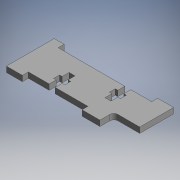
# Autodesk Inventor part: Part14
Saved by Autodesk Inventor 2019.2 (Build 232265000, 265)
## iProperties
Part Number: Part14
Material: Generic
Document SubType Name: Modeling
Designer: richard.girt
Mass: 2.90152 g
Surface Area: 27.0963 cm^2
Volume: 2.90152 cm^3
Density: 1 g/cm^3
Appearance: Default
Author: richard.girt
Autodesk Inventor part; units mm, degrees
ref_plane "YZ Plane" through (0, 0, 0) normal (1, 0, 0) x (0, 1, 0)
ref_plane "XZ Plane" through (0, 0, 0) normal (0, 1, 0) x (-1, 0, 0)
ref_plane "XY Plane" through (0, 0, 0) normal (0, 0, 1) x (1, 0, 0)
sketch "Sketch1" plane through (0, 0, 0) normal (0, 1, 0) x (-1, 0, 0)
  line L0 (-30, -12) -> (30, -12)
  line L1 (30, -12) -> (30, 12)
  line L2 (30, 12) -> (-30, 12)
  line L3 (-30, 12) -> (-30, -12)
  line L4 (-30, -12) -> (30, 12) construction
  line L5 (30, -12) -> (-30, 12) construction
  line L6 (25, -12) -> (-22, -12)
  line L7 (-22, -12) -> (-22, -9)
  line L8 (-22, -9) -> (25, -9)
  line L9 (25, -9) -> (25, -12)
  line L10 (22, 12) -> (-8, 12)
  line L11 (-8, 12) -> (-8, 9)
  line L12 (-8, 9) -> (22, 9)
  line L13 (22, 9) -> (22, 12)
  line L14 (-30, 12) -> (-17, 12)
  line L15 (-17, 12) -> (-17, 7)
  line L16 (-19, 5) -> (-30, 5)
  line L17 (-30, 5) -> (-30, 12)
  line L18 (11.75, -1) -> (8.25, -1)
  line L19 (8.25, -1) -> (8.25, 9)
  line L20 (8.25, 9) -> (11.75, 9)
  line L21 (11.75, 9) -> (11.75, -1)
  line L22 (11.75, -1) -> (8.25, 9) construction
  line L23 (8.25, -1) -> (11.75, 9) construction
  line L24 (12.8, 5.5) -> (7.2, 5.5)
  line L25 (7.2, 5.5) -> (7.2, 2.5)
  line L26 (7.2, 2.5) -> (12.8, 2.5)
  line L27 (12.8, 2.5) -> (12.8, 5.5)
  line L28 (12.8, 5.5) -> (7.2, 2.5) construction
  line L29 (7.2, 5.5) -> (12.8, 2.5) construction
  line L30 (-8.25, -9) -> (-11.75, -9)
  line L31 (-11.75, -9) -> (-11.75, 1)
  line L32 (-11.75, 1) -> (-8.25, 1)
  line L33 (-8.25, 1) -> (-8.25, -9)
  line L34 (-8.25, -9) -> (-11.75, 1) construction
  line L35 (-11.75, -9) -> (-8.25, 1) construction
  line L36 (-7.2, -2.5) -> (-12.8, -2.5)
  line L37 (-12.8, -2.5) -> (-12.8, -5.5)
  line L38 (-12.8, -5.5) -> (-7.2, -5.5)
  line L39 (-7.2, -5.5) -> (-7.2, -2.5)
  line L40 (-7.2, -2.5) -> (-12.8, -5.5) construction
  line L41 (-12.8, -2.5) -> (-7.2, -5.5) construction
  arc A0 (-19, 5) -> (-17, 7) centre (-19, 7) ccw
  point P0 (0, 0)
  point P1 (10, 4)
  point P2 (10, 4)
  point P3 (10, 9)
  point P4 (-10, -4)
  point P5 (-10, -4)
  point P6 (-10, 1)
  point P7 (-10, -9)
  dimension "d0" = 60
  dimension "d1" = 24
  dimension "d3" = 3
  dimension "d4" = 47
  dimension "d5" = 8
  dimension "d6" = 30
  dimension "d7" = 3
  dimension "d8" = 7
  dimension "d9" = 13
  dimension "d10" = 10
  dimension "d12" = 5.6
  dimension "d14" = 20
  dimension "d15" = 10
  dimension "d16" = 5.6
  dimension "d17" = 3.5
  dimension "d18" = 20
  dimension "d19" = 2
  dimension "d22" = 9
  dimension "d23" = 8
  dimension "d24" = 5
  dimension "d25" = 3
  constraints: 84 end point, 18 parallel, 15 midpoint, 8 horizontal, 8 perpendicular, 4 point on line, 2 point on circle, 2 tangent, 1 centre point
  measures "d0" distance of L0.start L0.end
  measures "d1" distance of L0.end L1.end
  measures "d3" distance of L8.end L6.start
  measures "d4" distance of L7.end L8.end
  measures "d5" distance between parallel lines of L1 L13
  measures "d6" distance between parallel lines of L11 L13
  measures "d7" distance of L12.end L10.start
  measures "d8" distance between parallel lines of L2 L16
  measures "d9" distance between parallel lines of L3 L15
  measures "d10" distance of L18.end L19.end
  measures "d12" distance of L24.start L24.end
  measures "d14" distance from line of point (10, 9) L1
  measures "d15" distance of L31.start L34.end
  measures "d16" distance of L36.start L37.start
  measures "d17" distance of L33.end L31.start
  measures "d18" distance from line of point (-10, -9) L3
  measures "d19" radius of A0
  measures "d22" distance between parallel lines of L11 L15
  measures "d23" distance between parallel lines of L3 L7
  measures "d24" distance between parallel lines of L1 L9
  measures "d25" distance of L37.start L38.start
extrude "Extrusion1" add sketch "Sketch1" along normal mid plane 2.8 contours L3 L16 A0 L15 L2 L11 L12 L19 L24 L25 L26 L18 L21 L27 L13 L1 L0 L9 L8 L33 L38 L39 L36 L32 L31 L37 L7
equation "\"d10\" = d15"
equation "\"d12\" = d16"
body "Solid1"
